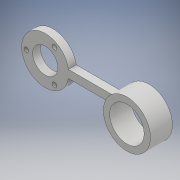
# Autodesk Inventor part: BarreCodeuseV2
Saved by Autodesk Inventor 2017 SP1 (Build 210196100, 196)
## iProperties
Part Number: BarreCodeuseV2
Material: Générique
Document SubType Name: Modeling
Designer: Sylvain
Density: 1 g/cm^3
Appearance: Par défaut
Author: Sylvain
## iProperties of the stored document BarreCodeuseV2_Impression 3D.ipt
Part Number: BarreCodeuseV2_Impression 3D
Material: Générique
Document SubType Name: Modeling
Designer: Sylvain
Density: 1 g/cm^3
Appearance: Par défaut
Author: Sylvain
Autodesk Inventor part; units mm, degrees
ref_plane "YZ Plane" through (0, 0, 0) normal (1, 0, 0) x (0, 1, 0)
ref_plane "XZ Plane" through (0, 0, 0) normal (0, 1, 0) x (-1, 0, 0)
ref_plane "XY Plane" through (0, 0, 0) normal (0, 0, 1) x (1, 0, 0)
sketch "Esquisse1" plane through (0, 0, 0) normal (0, 1, 0) x (-1, 0, 0)
  circle A0 centre (0, 0) radius 15
  circle A1 centre (0, 0) radius 8
  dimension "d0" = 30
  dimension "d1" = 16
  constraints: 2 centre point, 2 coincident
  measures "d0" diameter of A0
  measures "d1" diameter of A1
extrude "Extrusion1" add sketch "Esquisse1" along normal blind 5
sketch "Esquisse2" plane through (0, 5, 0) normal (0, 1, 0) x (1, 0, 0)
  circle A0 centre (0, 0) radius 15 projected
  point P0 (-12, 0)
  point P1 (6, -10.3923)
  point P2 (6, 10.3923)
  dimension "d4" = 12
  dimension "d7" = 360
  constraints: 7 other
  measures "d4" distance of A0.centre point (-12, 0)
hole "Perçage1" at (-12, 5, 0) at (6, 5, 10.3923) at (6, 5, -10.3923) direction (0, -1, 0) diameter 3 depth 8 tip angle 118
sketch "Esquisse3" plane through (0, 5, 0) normal (0, 1, 0) x (1, 0, 0)
  circle A0 centre (61.032, 0) radius 11
  circle A1 centre (61.032, 0) radius 15
  point P0 (0, 0)
  dimension "d16" = 61.032
  dimension "d17" = 22
  dimension "d18" = 30
  constraints: 2 centre point, 1 coincident
  measures "d16" distance of point (0, 0) A0.centre
  measures "d17" diameter of A0
  measures "d18" diameter of A1
extrude "Extrusion2" add sketch "Esquisse3" against normal blind 14
sketch "Esquisse4" plane through (0, 5, 0) normal (0, 1, 0) x (1, 0, 0)
  circle A0 centre (0, 0) radius 8 projected
  line L0 (8, 0) -> (48.6, 0)
  line L1 (48.6, 0) -> (48.6, 2.5)
  line L2 (48.6, 2.5) -> (8, 2.5)
  line L3 (8, 2.5) -> (8, 0)
  line L4 (8, 0) -> (48.6, 0)
  line L5 (48.6, 0) -> (48.6, -2.5)
  line L6 (48.6, -2.5) -> (8, -2.5)
  line L7 (8, -2.5) -> (8, 0)
  dimension "d21" = 2.5
  dimension "d22" = 2.5
  dimension "d23" = 40.6
  constraints: 16 end point, 4 parallel, 2 horizontal, 2 perpendicular, 1 horizontal alignment, 1 other
  measures "d21" distance between parallel lines of L2 L0
  measures "d22" distance between parallel lines of L6 L0
  measures "d23" distance between parallel lines of L3 L1
extrude "Extrusion3" add sketch "Esquisse4" against normal blind 5 contours L3 L2 L1 L0 | L0 L5 L6 L7
